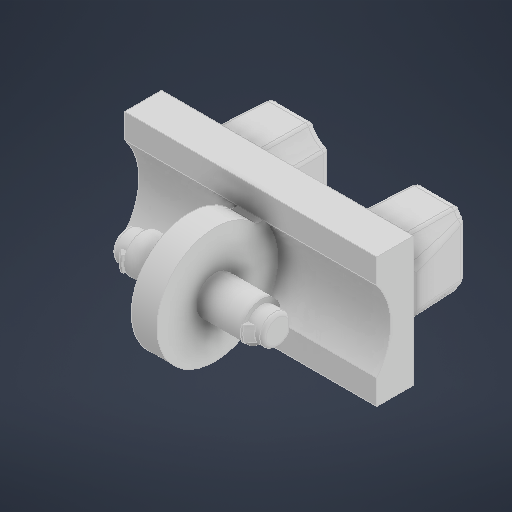
# Autodesk Inventor part: Lego connector piece
Saved by Autodesk Inventor 2027.1 (Build 311270010, 270A)
## iProperties
Created: 2020-11-13
Part Number: Lego connector piece
Material: Generic
Document SubType Name: Modeling
Designer: 164344
Density: 1 g/cm^3
Appearance: Default
Author: 164344
Autodesk Inventor part; units mm, degrees
ref_plane "YZ Plane" through (0, 0, 0) normal (1, 0, 0) x (0, 1, 0)
sketch "Sketch1" plane through (0, 0, 0) normal (0, 0, 1) x (1, 0, 0)
  line L0 (-7.6, -3.905) -> (7.6, -3.905)
  line L1 (7.6, -3.905) -> (7.6, 3.905)
  line L2 (7.6, 3.905) -> (-7.6, 3.905)
  line L3 (-7.6, 3.905) -> (-7.6, -3.905)
  line L4 (-7.6, -3.905) -> (7.6, 3.905) construction
  line L5 (7.6, -3.905) -> (-7.6, 3.905) construction
  point P0 (0, 0)
  dimension "d0" = 15.2
  dimension "d1" = 7.81
  constraints: 12 end point, 2 midpoint, 2 parallel, 1 horizontal, 1 perpendicular
  measures "d0" distance of L2.end L1.end
  measures "d1" distance of L1.end L0.end
extrude "Extrusion1" add sketch "Sketch1" along normal blind 2.22
sketch "Sketch2" plane through (7.6, -3.905, 0) normal (1, 0, 0) x (0, 0, -1)
  circle A0 centre (-5.22, 3.905) radius 3.85
  line L0 (-2.22, 0) -> (-2.22, 7.81) projected
  line L1 (0, 0) -> (0, 7.81) projected
  point P0 (0, 3.905)
  point P1 (0, 3.905)
  dimension "d4" = 7.7
  dimension "d5" = 3
  constraints: 1 centre point, 1 horizontal alignment, 1 midpoint
  measures "d4" diameter of A0
  measures "d5" distance from line of A0.centre L0
extrude "Extrusion2" cut sketch "Sketch2" against normal blind 15.2
ref_plane "Work Plane1" through (0, -3.905, 0) normal (-1, 0, 0) x (0, 0, 1)
sketch "Sketch3" plane through (0, -3.905, 0) normal (-1, 0, 0) x (0, 0, 1)
  arc A0 (2.62, 1.492) -> (2.62, 6.318) centre (5.1553, 3.905) ccw
  line L0 (2.22, 7.81) -> (2.22, 6.318) projected
  line L1 (2.22, 6.318) -> (2.62, 6.318)
  line L2 (2.22, 0) -> (2.22, 1.492) projected
  line L3 (2.22, 1.492) -> (2.62, 1.492)
  arc A1 (2.22, 6.318) -> (2.22, 1.492) centre (5.22, 3.905) ccw
  point P0 (0, 3.905)
  dimension "d9" = 7
  dimension "d10" = 0.4
  dimension "d11" = 0.4
  dimension "d12" = 3.85
  constraints: 4 end point, 4 point on circle, 2 centre point, 2 perpendicular
  measures "d9" diameter of A0
  measures "d10" distance of L0.end L1.end
  measures "d11" distance of L2.end L3.end
  measures "d12" radius of A1
extrude "Extrusion3" add sketch "Sketch3" along normal mid plane 1.55
sketch "Sketch4" plane through (0.775, -3.905, 0) normal (1, 0, 0) x (0, 0, -1)
  arc A0 (-2.62, 6.318) -> (-2.62, 1.492) centre (-5.1553, 3.905) ccw projected
  circle A1 centre (-5.1553, 3.905) radius 1.15
  point P0 (0, 3.905)
  dimension "d15" = 2.3
  constraints: 1 centre point, 1 coincident
  measures "d15" diameter of A1
extrude "Extrusion4" add sketch "Sketch4" along normal blind 2.8
sketch "Sketch5" plane through (3.575, 0, 5.1553) normal (1, 0, 0) x (0, 0, -1)
  arc A0 (0.6225, 0.65) -> (0.6225, -0.65) centre (0, 0) ccw
  line L0 (0.6225, 0.65) -> (0.6225, -0.65)
  circle A1 centre (0, 0) radius 1.15 projected
  point P0 (5.1553, 0)
  dimension "d18" = 1.8
  dimension "d19" = 1.3
  constraints: 2 end point, 2 point on circle, 1 centre point, 1 coincident, 1 vertical
  measures "d18" diameter of A0
  measures "d19" distance of L0.end L0.start
extrude "Extrusion5" add sketch "Sketch5" along normal blind 1 contours L0 A0
ref_plane "Work Plane2" through (4.075, 0, 5.1553) normal (1, 0, 0) x (0, 0, -1)
sketch "Sketch6" plane through (4.075, 0, 5.1553) normal (1, 0, 0) x (0, 0, -1)
  arc A0 (0.6225, 0.65) -> (0.6225, -0.65) centre (0, 0) ccw projected
  line L0 (0.6225, -0.65) -> (0.6225, 0.65) projected
  arc A1 (-1.1909, 0.4294) -> (-1.1723, -0.478) centre (0, 0) ccw
  line L1 (0.9885, 0.791) -> (0.9885, -0.791)
  line L2 (-0.7909, 0.4294) -> (-1.1909, 0.4294)
  line L3 (-0.7726, -0.4615) -> (-1.1723, -0.478)
  arc A2 (-0.7909, 0.4294) -> (-0.7726, -0.4615) centre (0, 0) ccw
  point P0 (5.1553, 0)
  dimension "d22" = 0.366
  dimension "d23" = 0.4
  dimension "d24" = 0.4
  constraints: 6 end point, 6 point on circle, 2 centre point, 1 horizontal
  measures "d22" radial gap between concentric circles of A0 A1
  measures "d23" distance of L2.end L2.start
  measures "d24" distance of L3.end L3.start
extrude "Extrusion6" add sketch "Sketch6" against normal blind 0.5 contours A0 L3 A1 L2
chamfer "Chamfer1" distance 0.35 angle 45 1 edges at (4.075, -0.026, 6.421)
fillet "Fillet1" radius 0.2 1 edges at (4.575, 0, 6.0553)
mirror "Mirror1" about plane through (0, -3.905, 0) normal (-1, 0, 0) of "Extrusion4", "Extrusion5", "Extrusion6", "Chamfer1", "Fillet1"
sketch "Sketch7" plane through (0, 0, 0) normal (0, 0, -1) x (-1, 0, 0)
  line L0 (5.75, 2.335) -> (3.05, 2.335)
  line L1 (2.05, 1.335) -> (2.05, -1.365)
  line L2 (3.05, -2.365) -> (5.75, -2.365)
  line L3 (6.75, -1.365) -> (6.75, 1.335)
  line L4 (7.6, -3.905) -> (-7.6, -3.905) projected
  line L5 (7.6, 3.905) -> (7.6, -3.905) projected
  arc A0 (6.75, -1.365) -> (5.75, -2.365) centre (7.1854, -2.8004) ccw
  arc A1 (3.05, -2.365) -> (2.05, -1.365) centre (1.6146, -2.8004) ccw
  arc A2 (5.75, 2.335) -> (6.75, 1.335) centre (7.1854, 2.7705) ccw
  arc A3 (2.05, 1.335) -> (3.05, 2.335) centre (1.6146, 2.7705) ccw
  line L6 (4.3354, -4.4212) -> (4.2283, -4.5283) construction
  line L7 (8.8212, -4.4212) -> (8.9283, -4.5283) construction
  line L8 (0, 5.6573) -> (0, -6.609) projected
  line L9 (-7.6, -3.905) -> (-7.6, 3.905) projected
  line L10 (7.6, 2.413) -> (7.6, -2.413) projected
  point P0 (0, 0)
  dimension "d33" = 4.7
  dimension "d35" = 1.5
  dimension "d36" = 1.5
  dimension "d37" = 1.5
  dimension "d39" = 2.7
  dimension "d40" = 1.5
  dimension "d41" = 2.7
  dimension "d42" = 2.7
  dimension "d43" = 2.7
  dimension "d44" = 1
  dimension "d45" = 1
  dimension "d46" = 1
  dimension "d47" = 1
  dimension "d48" = 1
  dimension "d49" = 1
  dimension "d50" = 1
  dimension "d51" = 1
  dimension "d57" = 4.7
  dimension "d58" = 1.54
  dimension "d59" = 1.85
  constraints: 12 end point, 8 point on circle, 4 centre point, 2 parallel, 1 horizontal, 1 perpendicular
  measures "d33" distance between parallel lines of L1 L3
  measures "d35" radius of A0
  measures "d36" radius of A1
  measures "d37" radius of A2
  measures "d39" distance of L0.end L0.start
  measures "d40" radius of A3
  measures "d41" distance of L1.start L1.end
  measures "d42" distance of L3.end L3.start
  measures "d43" distance of L2.start L2.end
  measures "d44" distance from line of L0.start L3
  measures "d45" horizontal distance of L3.end L0.start
  measures "d46" horizontal distance of L2.end L3.start
  measures "d47" horizontal distance of L2.end L3.start
  measures "d48" horizontal distance of L1.end L2.start
  measures "d49" horizontal distance of L1.end L2.start
  measures "d50" horizontal distance of L0.end L1.start
  measures "d51" horizontal distance of L1.start L0.end
  measures "d57" distance between parallel lines of L0 L2
  measures "d58" distance between parallel lines of L4 L2
  measures "d59" distance from line of L5 L0.start
extrude "Extrusion7" add sketch "Sketch7" along normal blind 4.85 draft -2
sketch "Sketch8" plane through (-7.6, 3.905, 0) normal (0, 1, 0) x (1, 0, 0)
  line L0 (0.8867, 1.05) -> (1.6867, 4.85)
  line L1 (1.6867, 4.85) -> (0.8867, 4.85)
  line L2 (0.8867, 4.85) -> (0.8867, 1.05)
  line L3 (1.9705, 4.85) -> (1.0194, 4.85) projected
  line L4 (15.2, 0) -> (0, 0) projected
  line L5 (0.85, 0) -> (1.0194, 4.85) projected
  point P0 (7.6, 0)
  dimension "d65" = 3.8
  dimension "d66" = 0.8
  dimension "d67" = 1.05
  dimension "d68" = 11.889
  dimension "d69" = 4.85
  dimension "d71" = 1.6867
  constraints: 6 end point, 1 perpendicular
  measures "d65" distance of L0.start L1.end
  measures "d66" distance of L1.end L0.end
  measures "d67" distance from line of L0.start L4
  measures "d68" angle of L0 L2
  measures "d69" distance between parallel lines of L4 L1
  measures "d71" horizontal distance of L4.end L0.end
extrude "Extrusion8" cut sketch "Sketch8" against normal through all
sketch "Sketch9" plane through (0, 0, -4.85) normal (0, 0, -1) x (-1, 0, 0)
  arc A0 (5.544, 0.985) -> (5.544, -1.015) centre (4.426, -0.015) ccw
  line L0 (5.75, -2.365) -> (3.05, -2.365) projected
  line L1 (2.05, -1.365) -> (2.05, 1.335) projected
  line L2 (5.544, -1.015) -> (5.544, 0.985)
  point P0 (0, 0)
  dimension "d74" = 3
  dimension "d75" = 2.35
  dimension "d76" = 2.376
  dimension "d77" = 2
  constraints: 2 end point, 2 point on circle, 1 centre point, 1 vertical
  measures "d74" diameter of A0
  measures "d75" distance from line of L0 A0.centre
  measures "d76" distance from line of L1 A0.centre
  measures "d77" distance of L2.end L2.start
extrude "Extrusion9" cut sketch "Sketch9" against normal blind 4.85
fillet "Fillet2" radius 0.5 8 edges at (-2.2194, -0.015, -4.85) (-4.4, 2.1657, -4.85) (-5.7515, 1.9157, -4.85) (-2.795, 1.59, -4.85) (-5.9133, -0.015, -4.85) (-5.7515, -1.9456, -4.85) (-4.4, -2.1956, -4.85) (-2.795, -1.62, -4.85)
fillet "Fillet3" radius 0.5 6 edges at (-6.0059, -1.6382, -4.4103) (-5.8215, -1.5678, -4.7392) (-6.3448, -1.4416, -2.8005) (-6.0059, 1.6083, -4.4103) (-5.8215, 1.5379, -4.7392) (-6.3448, 1.4117, -2.8005)
fillet "Fillet4" radius 0.2 12 edges at (-5.537, 2.0266, -4.7131) (-5.6955, 2.2602, -2.1438) (-3.263, 2.0266, -4.7131) (-3.1045, 2.2602, -2.1438) (-5.537, -2.0565, -4.7131) (-5.6955, -2.2901, -2.1438) (-2.3584, 1.1221, -4.7131) (-2.1249, 1.2806, -2.1438) (-2.3584, -1.152, -4.7131) (-2.1249, -1.3105, -2.1438) (-3.1045, -2.2901, -2.1438) (-3.263, -2.0565, -4.7131)
mirror "Mirror2" about plane through (0, -3.905, 0) normal (-1, 0, 0) of "Extrusion7", "Fillet2", "Extrusion9", "Fillet4", "Extrusion8", "Fillet3"
body "Solid1"
